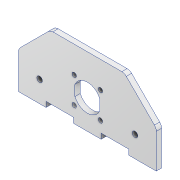
# Autodesk Inventor part: motor_wall
Saved by Autodesk Inventor 2020 (Build 240168000, 168)
## iProperties
Created: 2020-09-09
Part Number: motor_wall
Material: 알루미늄 6061
Document SubType Name: Sheet Metal
Designer: 이호석
Mass: 90.3904 g
Surface Area: 160.838 cm^2
Volume: 33.4779 cm^3
Density: 2.7 g/cm^3
Sheet Metal Rule: 기본값_mm
Appearance: 알루미늄 - 평지
Flat Pattern Width: 6.5 cm
Flat Pattern Length: 13 cm
Flat Pattern Area: 84.5 cm^2
Sheet Metal Width: 65.000 mm
Sheet Metal Length: 130.000 mm
Sheet Metal Area: 8450.000 mm^2
Author: 이호석
Autodesk Inventor part; units mm, degrees
ref_plane "YZ Plane" through (0, 0, 0) normal (1, 0, 0) x (0, 1, 0)
ref_plane "XZ Plane" through (0, 0, 0) normal (0, 1, 0) x (-1, 0, 0)
ref_plane "XY Plane" through (0, 0, 0) normal (0, 0, 1) x (1, 0, 0)
sketch "스케치1" plane through (0, 0, 0) normal (0, 0, 1) x (1, 0, 0)
  circle A0 centre (0, 0) radius 21.2
  line L0 (25, -22.5) -> (25, 27.5)
  line L1 (-25, 27.5) -> (-25, -22.5)
  circle A1 centre (0, 0) radius 22.3
  line L2 (25, 27.5) -> (-25, 27.5)
  line L3 (-11.7, 4.9396) -> (-11.7, -4.9396)
  arc A2 (-11.7, -4.9396) -> (11.7, -4.9396) centre (0, 0) ccw
  line L4 (11.7, -4.9396) -> (11.7, 4.9396)
  arc A3 (11.7, 4.9396) -> (-11.7, 4.9396) centre (0, 0) ccw
  circle A4 centre (12.3744, -12.3744) radius 2.1
  circle A5 centre (12.3744, 12.3744) radius 2.1
  circle A6 centre (-12.3744, 12.3744) radius 2.1
  circle A7 centre (-12.3744, -12.3744) radius 2.1
  line L5 (50, -22.5) -> (-50, -22.5)
  line L6 (50, -22.5) -> (50, -2.5)
  line L7 (50, -2.5) -> (25, 27.5)
  line L8 (-50, -22.5) -> (-50, -2.5)
  line L9 (-50, -2.5) -> (-25, 27.5)
  line L10 (-50, -22.5) -> (-65, -22.5)
  line L11 (50, -22.5) -> (65, -22.5)
  line L12 (65, -22.5) -> (65, -2.5)
  line L13 (-65, -22.5) -> (-65, -2.5)
  line L14 (-65, -2.5) -> (-25, 27.5)
  line L15 (25, 27.5) -> (65, -2.5)
  line L16 (-65, -22.5) -> (-65, 7.5)
  line L17 (65, -22.5) -> (65, 7.5)
  line L18 (25, -22.5) -> (25, 37.5)
  line L19 (-25, -22.5) -> (-25, 37.5)
  line L20 (-25, 37.5) -> (-65, 7.5)
  line L21 (-25, 37.5) -> (25, 37.5)
  line L22 (25, 37.5) -> (65, 7.5)
  line L23 (-25, 37.5) -> (-35, 37.5)
  line L24 (-35, 37.5) -> (-65, 7.5)
  line L25 (25, 37.5) -> (35, 37.5)
  line L26 (35, 37.5) -> (65, 7.5)
  dimension "d17" = 360
  dimension "d29" = 20
  dimension "d30" = 20
  dimension "d33" = 15
  dimension "d34" = 15
  dimension "d35" = 30
  dimension "d36" = 30
  dimension "d37" = 60
  dimension "d38" = 60
  dimension "d39" = 10
  dimension "d40" = 10
  measures "d29" distance of L5.start L6.end
  measures "d30" distance of L5.end L8.end
  measures "d33" distance of L5.end L10.end
  measures "d34" distance of L5.start L11.end
  measures "d35" distance of L10.end L16.end
  measures "d36" distance of L11.end L17.end
  measures "d37" distance of L0.start L18.end
  measures "d38" distance of L1.end L19.end
  measures "d39" distance of L19.end L23.end
  measures "d40" distance of L18.end L25.end
extrude "판1" add sketch "스케치1" along normal blind 5 contours A0 | L5 L1 L2 L0 | L0 L7 L6 L5 | L15 L12 L11 L6 L7 | L18 L22 L17 L15 | L2 L19 L21 L18 | L5 L8 L9 L1 | L9 L8 L10 L13 L14 | L14 L16 L20 L19 | L25 L26 L22 | L20 L24 L23 | A1
fillet "모서리 라운드2" radius 6 4 edges at (-35, 37.5, 2.5) (-65, 7.5, 2.5) (35, 37.5, 2.5) (65, 7.5, 2.5)
sketch "스케치2" plane through (0, 0, 5) normal (0, 0, 1) x (1, 0, 0)
  line L0 (-65, -22.5) -> (-65, 5.0147) projected
  line L1 (-65, -22.5) -> (-60, -22.5)
  line L2 (65, -22.5) -> (-65, -22.5) projected
  line L3 (65, -22.5) -> (60, -22.5)
  line L4 (60, -22.5) -> (30, -22.5)
  line L5 (30, -22.5) -> (30, 7.5)
  line L6 (30, 7.5) -> (60, 7.5)
  line L7 (60, 7.5) -> (60, -22.5)
  line L8 (-60, -22.5) -> (-30, -22.5)
  line L9 (-30, -22.5) -> (-30, 7.5)
  line L10 (-30, 7.5) -> (-60, 7.5)
  line L11 (-60, 7.5) -> (-60, -22.5)
  line L12 (-60, -22.5) -> (-45, -22.5)
  line L13 (-45, -22.5) -> (-45, -7.5)
  line L14 (60, -22.5) -> (45, -22.5)
  line L15 (45, -22.5) -> (45, -7.5)
  circle A0 centre (45, -7.5) radius 2.6
  circle A1 centre (-45, -7.5) radius 2.6
  point P0 (0, 0)
  dimension "d42" = 5
  dimension "d43" = 5
  dimension "d44" = 30
  dimension "d45" = 30
  dimension "d46" = 30
  dimension "d47" = 30
  dimension "d48" = 15
  dimension "d49" = 5.2
  dimension "d50" = 5.2
  constraints: 28 end point, 4 parallel, 3 perpendicular, 2 centre point, 2 coincident, 2 horizontal, 2 midpoint, 2 point on line, 1 vertical
  measures "d42" distance of L0.start L1.end
  measures "d43" distance of L2.start L3.end
  measures "d44" distance of L5.end L6.end
  measures "d45" distance of L4.end L5.end
  measures "d46" distance of L10.end L9.end
  measures "d47" distance of L9.end L8.end
  measures "d48" distance of L3.end L14.end
  measures "d49" diameter of A0
  measures "d50" diameter of A1
extrude "돌출1" cut sketch "스케치2" against normal through all contours A0 | A1
sketch "스케치3" plane through (0, 0, 5) normal (0, 0, 1) x (1, 0, 0)
  line L0 (65, -22.5) -> (-65, -22.5) projected
  line L1 (-65, -22.5) -> (65, -22.5)
  line L2 (65, -22.5) -> (65, -27.5)
  line L3 (65, -27.5) -> (-65, -27.5)
  line L4 (-65, -27.5) -> (-65, -22.5)
  line L5 (-65, -22.5) -> (-39, -22.5)
  line L6 (-39, -22.5) -> (-13, -22.5)
  line L7 (-13, -22.5) -> (13, -22.5)
  line L8 (13, -22.5) -> (39, -22.5)
  line L9 (39, -22.5) -> (65, -22.5)
  line L10 (-39, -22.5) -> (-39, -27.5)
  line L11 (-13, -22.5) -> (-13, -27.5)
  line L12 (13, -22.5) -> (13, -27.5)
  line L13 (39, -22.5) -> (39, -27.5)
  point P0 (0, 0)
  dimension "d53" = 130
  dimension "d54" = 5
  dimension "d55" = 26
  dimension "d56" = 26
  dimension "d57" = 26
  dimension "d58" = 26
  dimension "d59" = 26
  constraints: 26 end point, 8 point on line, 3 parallel, 3 perpendicular, 1 collinear, 1 horizontal, 1 vertical
  measures "d53" distance of L2.end L3.end
  measures "d54" distance of L1.end L2.end
  measures "d55" distance of L0.end L5.end
  measures "d56" distance of L5.end L6.end
  measures "d57" distance of L6.end L7.end
  measures "d58" distance of L7.end L8.end
  measures "d59" distance of L8.end L1.end
extrude "돌출2" add sketch "스케치3" against normal blind 5 contours L2 L3 L13 L0 | L12 L3 L11 L0 | L10 L3 L4 L0
equation "\"TransitionRadius\" = BendRadius"
equation "\"BendRadius\" = 5"
